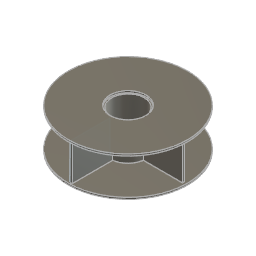
3D SPOOL (Autodesk Fusion 360 design; units mm, degrees)
part number: 2026-06-12-14-53-29-503
Autodesk Fusion 360 part; units mm, degrees
sketch "Sketch1" plane through (0, 0, 0) normal (0, 1, 0) x (1, 0, 0)
  circle A0 centre (0, 0) radius 100
  dimension "d1" = 200
  constraint coincident A0.centre origin
  measures "d1" diameter of A0
extrude "Extrude1" add sketch "Sketch1" along normal blind 1 makes body 1
extrude "Extrude2" add 1 faces at (-27.1036, 1, 4.9681) along direction (0, 1, 0) blind 2 on bodies 1 bodies 1
sketch "Sketch2" plane through (0, 3, 0) normal (0, 1, 0) x (-1, 0, 0)
  circle A0 centre (0, 0) radius 100
  circle A1 centre (0, 0) radius 30
  dimension "d6" = 60
  constraint coincident A0.centre A1.centre
  measures "d6" diameter of A1
extrude "Extrude3" add sketch "Sketch2" along normal blind 60 contours A1 bodies 1
sketch "Sketch3" plane through (0, 63, 0) normal (0, 1, 0) x (-1, 0, 0)
  circle A0 centre (0, 0) radius 30
  circle A1 centre (0, 0) radius 100
  circle A2 centre (0, 0) radius 27.5
  dimension "d9" = 200
  dimension "d10" = 55
  constraint coincident A0.centre A1.centre
  measures "d9" diameter of A1
  measures "d10" diameter of A2
extrude "Extrude4" cut sketch "Sketch3" against normal blind 80 contours A2 bodies 1
sketch "Sketch4" plane through (0, 0, 0) normal (0, 1, 0) x (1, 0, 0)
sketch "Sketch5" plane through (0, 63, 0) normal (0, 1, 0) x (-1, 0, 0)
  circle A0 centre (0, 0) radius 27.5
  circle A1 centre (0, 0) radius 30
  circle A2 centre (0, 0) radius 100
  dimension "d13" = 200
  constraint coincident A0.centre A1.centre
  measures "d13" diameter of A2
extrude "Extrude5" add sketch "Sketch5" along normal blind 3 separate body contours A2 makes body 2
combine "Combine1" operation add target body 2 tool bodies 1
sketch "Sketch6" plane through (0, 0, 0) normal (0, 0, 1) x (1, 0, 0)
  line L0 (30, 63) -> (95, 63)
  line L1 (95, 63) -> (95, 3)
  line L2 (95, 3) -> (30, 3)
  line L3 (30, 3) -> (30, 63)
  constraint horizontal L0
  constraint perpendicular L0 L1
  constraint perpendicular L1 L2
extrude "Extrude6" add sketch "Sketch6" along normal blind 4 separate body makes body 3
sketch "Sketch7" plane through (0, 0, 0) normal (1, 0, 0) x (0, 0, -1)
  line L0 (30, 63) -> (95, 63)
  line L1 (95, 63) -> (95, 3)
  line L2 (95, 3) -> (30, 3)
  line L3 (30, 3) -> (30, 63)
  constraint horizontal L0
  constraint perpendicular L0 L1
  constraint perpendicular L1 L2
  constraint perpendicular L0 L3
extrude "Extrude7" add sketch "Sketch7" along normal blind 4 separate body makes body 4
sketch "Sketch8" plane through (0, 0, 0) normal (0, 0, 1) x (1, 0, 0)
  line L0 (-30, 63) -> (-97, 63)
  line L1 (-97, 63) -> (-97, 3)
  line L2 (-97, 3) -> (-30, 3)
  line L3 (-30, 3) -> (-30, 63)
  constraint horizontal L0
  constraint perpendicular L0 L1
  constraint perpendicular L1 L2
  constraint perpendicular L2 L3
extrude "Extrude8" add sketch "Sketch8" along normal blind 4 separate body makes body 5
sketch "Sketch9" plane through (0, 0, 0) normal (1, 0, 0) x (0, 0, -1)
  line L0 (-30, 63) -> (-97, 63)
  line L1 (-97, 63) -> (-97.5, 3)
  line L2 (-97.5, 3) -> (-30, 3)
  line L3 (-30, 3) -> (-30, 63)
  constraint horizontal L0
  constraint parallel L0 L2
extrude "Extrude9" add sketch "Sketch9" along normal blind 4 separate body makes body 6
sketch "Sketch10" plane through (0, 0, 0) normal (-1, 0, 0) x (0, 0, 1)
  line L0 (30, 63) -> (30, 3)
  line L1 (30, 3) -> (97.5, 3)
  line L2 (97.5, 3) -> (97, 63)
  line L3 (97, 63) -> (30, 63)
